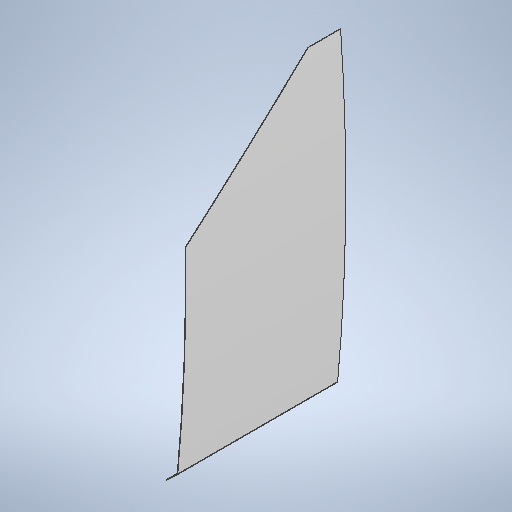
# Autodesk Inventor part: MSC 025 sheet left-right board withers 1
Saved by Autodesk Inventor 2025 (Build 290162010, 162A)
## iProperties
Created: 2024-04-18
Part Number: MSC 025 sheet left-right board withers 1
Material: AISI304
Document SubType Name: Sheet Metal
Designer: admin
Stock Number: МОО 025 лист левый-правый борт холка 1
Mass: 48027.3 g
Surface Area: 40202.8 cm^2
Volume: 6003.41 cm^3
Density: 8 g/cm^3
Flat Pattern Width: 98 cm
Flat Pattern Length: 197.929 cm
Flat Pattern Area: 19397 cm^2
Sheet Metal Rule: Default_mm
Sheet Metal Width: 980,000 mm
Sheet Metal Length: 1979,289 mm
Sheet Metal Area: 1939703,615 mm^2
Appearance: Default
Author: admin
Autodesk Inventor part; units mm, degrees
ref_plane "YZ Plane" through (0, 0, 0) normal (1, 0, 0) x (0, 1, 0)
ref_plane "XZ Plane" through (0, 0, 0) normal (0, 1, 0) x (-1, 0, 0)
ref_plane "XY Plane" through (0, 0, 0) normal (0, 0, 1) x (1, 0, 0)
sketch "Sketch1" plane through (0, 0, 0) normal (0, 0, 1) x (1, 0, 0)
  line L0 (-750, 0) -> (750, 0) construction
  line L1 (750, 0) -> (750, -2700) construction
  line L2 (750, -2700) -> (-750, -2700) construction
  line L3 (-750, -2700) -> (-750, 0) construction
  line L4 (800, 50) -> (-800, 50) construction
  line L5 (-800, 50) -> (-800, -2750) construction
  line L6 (-800, -2750) -> (800, -2750) construction
  line L7 (800, -2750) -> (800, 50) construction
  line L8 (-850, 100) -> (850, 100) construction
  line L9 (850, 100) -> (850, -2800) construction
  line L10 (850, -2800) -> (-850, -2800) construction
  line L11 (-850, -2800) -> (-850, 100) construction
  line L12 (-750, -2100) -> (750, -2100) construction
  line L13 (115.485997, -2697.8227) -> (682.456682, -2163.637569) construction
  arc A0 (750, -2100) -> (750.178737, -2098.125829) centre (-10250, -1050) ccw construction
  arc A1 (748.630029, -2101.290751) -> (750.178737, -2098.125829) centre (745.201281, -2097.651564) ccw
  arc A2 (110, -2700) -> (115.485997, -2697.8227) centre (110, -2692) ccw construction
  line L14 (684.513931, -2165.821082) -> (682.456682, -2163.637569) construction
  arc A3 (750, 0) -> (0, 50) centre (0, -5600) ccw construction
  line L15 (0, 100) -> (0, 50) construction
  line L16 (0, -2700) -> (0, -2698.220626) construction
  line L17 (0, 47) -> (0, 0) construction
  line L18 (682.456682, -2163.637569) -> (748.630029, -2101.290751)
  arc A4 (750.178737, -2098.125829) -> (768.550013, -216.9) centre (-10250, -1050) ccw
  line L19 (748.630029, -2101.290751) -> (750, -2100) construction
  line L20 (768.550013, -216.9) -> (750, 0) construction
  point P0 (0, -2750)
  dimension "d135" = 1500
  dimension "d136" = 2700
  dimension "d137" = 2100
  dimension "d138" = 5
  dimension "d139" = 8
  dimension "d140" = 50
  dimension "d141" = 50
  dimension "d142" = 110
  dimension "d143" = 92.8
  dimension "d144" = 216.9
  measures "d135" distance of L3.end L20.end
  measures "d136" distance of L20.end L1.end
  measures "d137" distance between parallel lines of L12 L0
  measures "d138" radius of A1
  measures "d139" radius of A2
  measures "d140" distance between parallel lines of L4 L8
  measures "d141" distance between parallel lines of L0 L4
  measures "d142" distance from line of L16 A2.centre
  measures "d143" distance of L12.end L18.start
  measures "d144" vertical distance of L20.start L20.end
contour flange "Contour Flange2" sketch "Sketch1" thickness 3 bend radius 3 width 980 along (0, 0, 1) mid plane no both sides no wall seen from (715.543355, -2132.46416, 0) lies toward (0.6857497, -0.7278375, 0) curves L18 A1 A4
bend "Bend2"
corner "Corner2"
sketch "Sketch2" plane through (0, 0, 0) normal (1, 0, 0) x (0, 1, 0)
  line L0 (-2099.15936, 980) -> (-2099.15936, 0)
  line L1 (-2099.15936, 0) -> (-215.885377, 0)
  line L2 (-215.885377, 0) -> (-215.885377, 980)
  line L3 (-2099.15936, 980) -> (-215.885377, 980)
  line L4 (-215.885377, 198.209643) -> (-871.885377, 980)
  line L5 (-215.885377, 781.790357) -> (-871.885377, 0)
  point P0 (0, 0)
  dimension "d129" = 40
  dimension "d134" = 656
  constraints: 4 end point, 4 point on line, 1 equal length, 1 vertical alignment
  measures "d129" angle of L2 L4
  measures "d134" distance from line of L2 L4.end
extrude "Extrusion2" cut sketch "Sketch2" along normal through all both and the other way through all contours L3 L2 L5 L4 | L5 L2 L4
sketch "Sketch5" plane through (749.1768, -2100.77463, 980) normal (-0.6852958, 0.7282648, 0) x (0.7282648, 0.6852958, 0)
  line L0 (-66.148757, 29.818011) -> (-66.148757, 287.62302) construction
  line L1 (-66.148757, 287.62302) -> (-28.600579, 287.62302) construction
  line L2 (-28.600579, 287.62302) -> (-28.600579, 29.818011) construction
  line L3 (-28.600579, 29.818011) -> (-66.148757, 29.818011) construction
  point P0 (894.052911, 980)
  constraints: 2 other
mark "Mark4"
equation "\"d36\" = Thickness"
equation "\"d37\" = BendReliefWidth"
equation "\"d38\" = BendReliefDepth"
equation "\"d39\" = MinimumRemnant"
equation "\"d40\" = TransitionRadius"
equation "\"d42\" = BendRadius"
equation "\"d44\" = CornerReliefSize"
equation "\"d45\" = GapSize"
equation "\"d46\" = JacobiRadiusSize"
equation "\"BendRadius\" = Thickness"
equation "\"BendReliefWidth\" = Thickness"
equation "\"BendReliefDepth\" = 0.5 * Thickness"
equation "\"CornerReliefSize\" = 4 * Thickness"
equation "\"MinimumRemnant\" = 2 * Thickness"
equation "\"TransitionRadius\" = BendRadius"
equation "\"JacobiRadiusSize\" = BendRadius"
equation "\"GapSize\" = Thickness"
equation "\"Thickness\" = 3"
body "Solid3"
